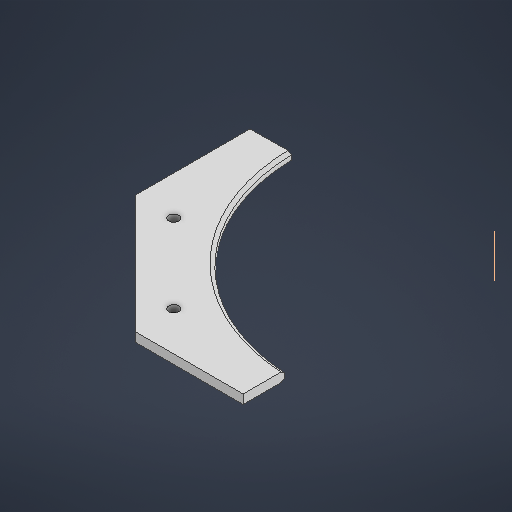
# Autodesk Inventor part: шутер на подш
Saved by Autodesk Inventor 2026.2 (Build 302298000, 298)
## iProperties
Created: 2026-01-20
Part Number: шутер на подш
Material: Типовые
Document SubType Name: Modeling
Designer: Phantom
Density: 1 g/cm^3
Appearance: По умолчанию
Author: Phantom
Autodesk Inventor part; units mm, degrees
ref_plane "YZ Plane" through (0, 0, 0) normal (1, 0, 0) x (0, 1, 0)
ref_plane "XY Plane" through (0, 0, 0) normal (0, 0, 1) x (1, 0, 0)
sketch "Эскиз1" plane through (0, 0, 0) normal (0, 0, 1) x (1, 0, 0)
  line L0 (0, 0) -> (-13, 0)
  line L1 (0, 0) -> (0, -7)
  line L2 (0, -7) -> (-13, -7)
  line L3 (0, -3.5) -> (-10, -3.5)
  arc A0 (-13, -6) -> (-13, -1) centre (-12.5417, -3.5) ccw
  arc A1 (-12.9459, -5.7049) -> (-12.9459, -1.2951) centre (-12.5417, -3.5) ccw
  line L4 (-10, -3.5) -> (-13.6021, -3.5)
  line L5 (-13.6021, -1.5) -> (-10, -1.5)
  line L6 (-10, -1.5) -> (0, -1.5)
  line L7 (-13.6021, -5.5) -> (-10, -5.5)
  line L8 (-10, -5.5) -> (0, -5.5)
  line L9 (-13.6021, -2.5) -> (-10, -2.5)
  line L10 (-10, -2.5) -> (0, -2.5)
  line L11 (-13.6021, -4.5) -> (-10, -4.5)
  line L12 (-10, -4.5) -> (0, -4.5)
  line L13 (-11.5292, -1.5) -> (-12.0292, -1.5)
  line L14 (-12.0292, -1.5) -> (-10.5354, -2.5)
  line L15 (-12.0292, -5.5) -> (-10.5354, -4.5)
  line L16 (-13.6021, -1.5) -> (-13.6021, -5.5)
  point P0 (-10.5354, -4.5)
  dimension "d0" = 13
  dimension "d1" = 7
  dimension "d2" = 1
  dimension "d3" = 1
  dimension "d4" = 10
  dimension "d5" = 0.3
  dimension "d6" = 2
  dimension "d7" = 2
  dimension "d8" = 1
  dimension "d9" = 1
  dimension "d10" = 0.5
  constraints: 34 end point, 7 point on circle, 3 horizontal, 3 point on line, 2 centre point, 2 symmetric about line, 2 vertical, 1 midpoint, 1 perpendicular, 4 other
  measures "d0" distance of L0.start L0.end
  measures "d1" distance of L0.start L1.end
  measures "d2" distance of L2.end A0.start
  measures "d3" distance of L0.end A0.end
  measures "d4" distance of L3.start L3.end
  measures "d5" radial gap between concentric circles of A0 A1
  measures "d6" distance between parallel lines of L4 L5
  measures "d7" distance between parallel lines of L4 L7
  measures "d8" distance between parallel lines of L4 L9
  measures "d9" distance between parallel lines of L4 L11
  measures "d10" distance of L13.start L13.end
sketch "Эскиз2" plane through (0, 0, 0) normal (0, 1, 0) x (-1, 0, 0)
  line L0 (13, 0) -> (10, 0) projected
  line L1 (10, 0) -> (-76.5, 0)
  circle A0 centre (-76.5, 0) radius 86.5
  point P0 (0, 0)
  dimension "d13" = 86.5
  constraints: 2 end point, 1 coincident, 1 horizontal, 1 horizontal alignment, 2 other
  measures "d13" distance of L0.end L1.end
sweep "Сдвиг1" add profiles "Эскиз1" path "Эскиз2" path curves A0 contours L4 L16 L9 A1 | A1 L11 L16 L4 | L9 L16 L5 L14 | L15 L7 L16 L11
sketch "Эскиз3" plane through (0, 0, 0) normal (0, 1, 0) x (-1, 0, 0)
  circle A0 centre (-76.5, 0) radius 90.1021 projected
  line L0 (28.5, -105) -> (-181.5, -105)
  line L1 (-181.5, -105) -> (-181.5, 105)
  line L2 (-181.5, 105) -> (28.5, 105)
  line L3 (28.5, 105) -> (28.5, -105)
  line L4 (28.5, -105) -> (-181.5, 105) construction
  line L5 (-181.5, -105) -> (28.5, 105) construction
  circle A1 centre (-76.5, 0) radius 87.0354 projected
  point P0 (0, 0)
  dimension "d16" = 210
  dimension "d17" = 210
  constraints: 12 end point, 2 midpoint, 2 parallel, 1 horizontal, 1 perpendicular
  measures "d16" distance of L1.end L2.end
  measures "d17" distance of L0.end L1.end
extrude "Выдавливание2" add sketch "Эскиз3" against normal up to surface (5.5 mm away) contours L0 L1 L2 L3
sketch "Эскиз4" plane through (0, 0, 0) normal (0, 1, 0) x (1, 0, 0)
  line L0 (-28.5, -105) -> (181.5, -105) projected
  line L1 (181.5, -105) -> (181.5, 105) projected
  line L2 (181.5, 105) -> (-28.5, 105) projected
  line L3 (-28.5, 105) -> (-28.5, -105) projected
  circle A0 centre (76.5, 0) radius 90.1021 projected
  point P0 (0, 0)
extrude "Выдавливание3" cut sketch "Эскиз4" against normal up to surface (1.5 mm away)
sketch "Эскиз5" plane through (-28.5, -1.5, -105) normal (0, 1, 0) x (1, 0, 0)
  line L0 (0, 0) -> (210, 0) projected
  line L1 (0, -210) -> (0, 0) projected
  line L2 (210, -210) -> (0, -210) projected
  line L3 (210, 0) -> (210, -210) projected
  circle A0 centre (105, -105) radius 88.5292 projected
  line L4 (0, -158.0794) -> (51.9206, -210)
  line L5 (42.4004, -167.5996) -> (25.9603, -184.0397)
  line L6 (0, -141.1088) -> (68.8912, -210)
  circle A1 centre (17.2229, -158.3318) radius 2.25
  circle A2 centre (51.6682, -192.7771) radius 2.25
  point P0 (28.5, -105)
  dimension "d22" = 45
  dimension "d24" = 12
  dimension "d26" = 4.5
  dimension "d34" = 99.779
  dimension "d41" = 24.3565
  constraints: 6 end point, 5 point on line, 2 centre point, 1 midpoint, 1 parallel, 1 symmetric about line, 4 other
  measures "d22" angle of L4 L1
  measures "d24" distance between parallel lines of L4 L6
  measures "d26" diameter of A1
  measures "d34" distance from line of point (105, -105) L6
  measures "d41" distance from line of L5 A1.centre
extrude "Выдавливание4" cut sketch "Эскиз5" against normal blind 10 contours L4 L2 L1 | A1 L6 | L6 A1 | A2 L6 | L6 A2
sketch "Эскиз6" plane through (23.4206, -1.5, 105) normal (0, 1, 0) x (1, 0, 0)
  line L0 (-51.9206, 210) -> (-51.9206, 51.9206) projected
  line L1 (-51.9206, 102.3308) -> (158.0794, 105)
  line L2 (158.0794, 210) -> (158.0794, 0) projected
  line L3 (-51.9206, 210) -> (158.0794, 210) projected
  line L4 (47.4225, 210) -> (47.4225, 0)
  line L5 (158.0794, 0) -> (0, 0) projected
  line L6 (0, 210) -> (-57.5775, 152.4225) projected
  line L7 (-57.5775, 57.5775) -> (-57.5775, 152.4225) projected
  line L8 (-57.5775, 57.5775) -> (0, 0) projected
  line L9 (94.845, 0) -> (0, 0) projected
  line L10 (94.845, 0) -> (152.4225, 57.5775) projected
  line L11 (152.4225, 152.4225) -> (152.4225, 57.5775) projected
  line L12 (152.4225, 152.4225) -> (94.845, 210) projected
  line L13 (0, 210) -> (94.845, 210) projected
  circle A0 centre (-43.7762, 60.7467) radius 2.25 projected
  circle A1 centre (47.4225, 105) radius 89.5292 projected
  point P0 (-23.4206, 105)
  point P1 (-51.9206, 51.9206)
  point P2 (-51.9206, 158.0794)
  point P3 (47.4225, 103.5935)
  point P4 (152.4225, 57.5775)
  point P5 (152.4225, 152.4225)
  point P6 (94.845, 210)
  point P7 (-51.9206, 51.9206)
  point P8 (152.4225, 104.9281)
  point P9 (0, 0)
  constraints: 4 end point, 2 point on line, 4 other
extrude "Выдавливание5" cut sketch "Эскиз6" against normal blind 10 contours L0 L6 L3 L4 A1 L1 | L0 L3 L6 | A1 L4 L1 | L4 A1 L1 | L1 A1 L4 | L4 L3 L12 L11 L1 A1 | A1 L1 L11 L10 L5 L4 | L10 L11 L1 L2 L5 | L3 L2 L1 L11 L12 picked at (43.0991, 163.9025) picked at (51.6696, 163.9135) picked at (106.793, 100.114)
